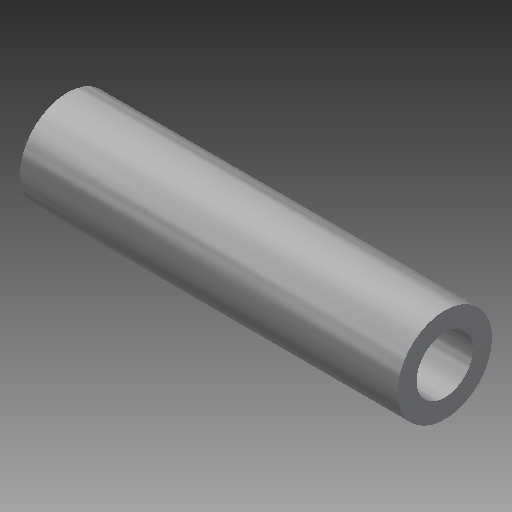
# Autodesk Inventor part: Shaft
Saved by Autodesk Inventor 2019 (Build 230136000, 136)
## iProperties
Created: 2019-11-01
Part Number: Shaft
Material: Steel
Document SubType Name: Modeling
Designer: Mark
Density: 1 g/cm^3
Appearance: Steel
CustomPartVersion: 1
Author: Mark
Autodesk Inventor part; units mm, degrees
ref_plane "Start Plane" through (0, 0, 0) normal (1, 0, 0) x (0, 1, 0)
ref_plane "XZ Plane" through (0, 0, 0) normal (0, 1, 0) x (-1, 0, 0)
ref_plane "XY Plane" through (0, 0, 0) normal (0, 0, 1) x (1, 0, 0)
sketch "Main Sketch" plane through (0, 0, 0) normal (0, 0, 1) x (1, 0, 0)
  line L0 (0, 0) -> (40, 0)
  line L1 (0, 3) -> (0, 5)
  line L2 (40, 5) -> (40, 3)
  line L3 (0, 5) -> (40, 5)
  line L4 (12, 3) -> (12, 0)
  line L5 (0, 3) -> (12, 3)
  line L6 (28, 3) -> (28, 0)
  line L7 (40, 3) -> (28, 3)
  line L8 (12, 0) -> (28, 0)
  dimension "d3" = 10
  dimension "d4" = 6
  dimension "d5" = 6
  constraints: 18 end point, 6 horizontal, 4 vertical
  measures "d3" diameter of L3 L0
  measures "d4" diameter of L5 L0
  measures "d5" diameter of L7 L0
revolve "Revolution1" add sketch "Main Sketch" angle 360 about axis through (0, 0, 0) along (1, 0, 0)
body "Solid1"
